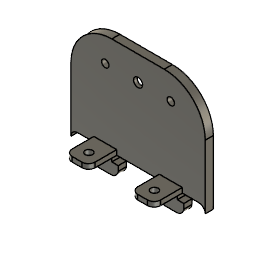
rodSupport (Autodesk Fusion 360 design; units mm, degrees)
part number: 2026-01-29-15-29-34-594
Autodesk Fusion 360 part; units mm, degrees
sketch "Sketch5" plane through (0, 0, 0) normal (0, 0, 1) x (1, 0, 0)
  line L0 (-41, -2.5) -> (41, -2.5)
  line L1 (41, -2.5) -> (41, 2.5)
  line L2 (41, 2.5) -> (-41, 2.5)
  line L3 (-41, 2.5) -> (-41, -2.5)
  line L4 (-41, -2.5) -> (41, 2.5) construction
  line L5 (41, -2.5) -> (-41, 2.5) construction
  line L6 (-37, 2.5) -> (-37, -2.5)
  line L7 (0, 2.5) -> (0, -2.5) construction
  line L8 (37, 2.5) -> (37, -2.5)
  line L9 (-10, -2.5) -> (10, -2.5) construction
  line L10 (23.95, -2.5) -> (16.05, -2.5)
  line L11 (16.05, -2.5) -> (16.05, 2.5)
  line L12 (16.05, 2.5) -> (23.95, 2.5)
  line L13 (23.95, 2.5) -> (23.95, -2.5)
  line L14 (-23.95, 2.5) -> (-23.95, -2.5)
  line L15 (-16.05, -2.5) -> (-16.05, 2.5)
  line L16 (-20, -2.5) -> (-20, 2.5) construction
  line L17 (20, -2.5) -> (20, 2.5) construction
  line L18 (-27, -2.5) -> (-13, -2.5)
  line L19 (-13, -2.5) -> (-13, -19.75)
  line L20 (-13, -19.75) -> (-27, -19.75)
  line L21 (-27, -19.75) -> (-27, -2.5)
  circle A0 centre (-20, -12.5) radius 2.25
  circle A1 centre (20, -12.5) radius 2.25
  line L22 (13, -19.75) -> (27, -19.75)
  line L23 (27, -19.75) -> (27, -2.5)
  line L24 (13, -2.5) -> (13, -19.75)
  dimension "d29" = 5
  dimension "d30" = 4
  dimension "d55" = 7.9
  dimension "d64" = 3.95
  dimension "d65" = 3.95
  dimension "d93" = 74
  dimension "d94" = 4
  dimension "d104" = 40
  dimension "d105" = 14
  dimension "d106" = 17.25
  dimension "d107" = 4.5
  dimension "d120" = 10
  constraint horizontal L0
  constraint perpendicular L0 L1
  constraint parallel L0 L2
  constraint parallel L1 L3
  constraint coincident L4 origin
  constraint coincident L5 origin
  constraint coincident L2 L6.start
  constraint coincident L0 L6.end
  constraint perpendicular L0 L6
  constraint midpoint L2 L7.start
  constraint midpoint L0 L7.end
  constraint symmetric L6.start L7 L8.start
  constraint symmetric L6.end L7 L8.end
  constraint horizontal L9
  constraint coincident L0 L9.start
  constraint horizontal L10
  constraint vertical L11
  constraint horizontal L12
  constraint vertical L13
  constraint coincident L0 L10.start
  constraint symmetric L7 L10.start L14.end
  constraint symmetric L7 L10.end L15.start
  constraint symmetric L7 L11.end L15.end
  constraint symmetric L7 L12.end L14.start
  constraint coincident L0 L16.start
  constraint coincident L2 L16.end
  constraint perpendicular L2 L16
  constraint symmetric L7 L16.start L17.start
  constraint symmetric L7 L16.end L17.end
  constraint coincident L2 L15.end
  constraint horizontal L18
  constraint vertical L19
  constraint horizontal L20
  constraint vertical L21
  constraint coincident L0 L18.start
  constraint midpoint L16.start L18
  constraint symmetric L7 L18.start L23.end
  constraint symmetric L7 L18.end L24.start
  constraint symmetric L7 L19.end L22.start
  constraint symmetric L7 L20.end L22.end
  constraint symmetric L7 A0 A1
  constraint vertical L16.start A0.centre
  measures "d29" distance of L0.end L1.end
  measures "d30" distance of L3 L6
  measures "d55" distance of L10.start L10.end
  measures "d64" distance of L14 L16
  measures "d65" distance of L15 L16
  measures "d93" distance of L6 L8
  measures "d94" distance of L1 L8
  measures "d104" distance of L16 L17
  measures "d105" distance of L18.start L18.end
  measures "d106" distance of L18.start L20.end
  measures "d107" diameter of A0
  measures "d120" distance of L18 A0.centre
sketch "Sketch6" plane through (0, 0, 0) normal (0, 1, 0) x (1, 0, 0)
  circle A0 centre (0, -45) radius 2.75
  line L0 (0, -56.6756) -> (0, 40) construction
  line L1 (-20, 40) -> (-20, 0) construction
  line L2 (20, 40) -> (20, 0) construction
  line L3 (20, 40) -> (20, 0) construction
  circle A1 centre (0, -45) radius 8.1
  line L4 (37.9681, -45) -> (-37.9681, -45) construction
  circle A2 centre (-20, -45) radius 2.25
  circle A3 centre (20, -45) radius 2.25
  point P0 (0, -45)
  point P1 (0, -60)
  point P2 (0, -56.6756)
  point P3 (0, 40)
  point P4 (-20, 16)
  point P5 (20, 16)
  point P6 (-20, 12)
  point P7 (-20, 5)
  point P8 (20, 16)
  point P9 (20, 5)
  point P10 (-20, 24)
  point P11 (20, 24)
  point P12 (-24.75, 0)
  point P13 (-37, 0)
  point P14 (20, 24)
  point P15 (20, 12)
  point P16 (37, 0)
  point P17 (20, 16)
  point P18 (24.75, 0)
  point P19 (20, 5)
  point P20 (0, -3)
  dimension "d35" = 5.5
  dimension "d36" = 40
  dimension "d45" = 20
  dimension "d46" = 20
  dimension "d48" = 40
  dimension "d49" = 12
  dimension "d50" = 5
  dimension "d51" = 16
  dimension "d52" = 8
  dimension "d53" = 16
  dimension "d54" = 12.25
  dimension "d77" = 15
  dimension "d99" = 16.2
  dimension "d103" = 45
  dimension "d108" = 3
  dimension "d115" = 4.5
  dimension "d116" = 20
  constraint vertical P1 L0.start
  constraint vertical P0 P1
  constraint coincident P0 A0.centre
  constraint coincident P2 L0.start
  constraint coincident P3 L0.end
  constraint vertical L0
  constraint horizontal P4 P17
  constraint horizontal P3 L1.start
  constraint vertical P4 L1.start
  constraint coincident L1 P6
  constraint coincident L1 P7
  constraint symmetric P4 L0 P17
  constraint symmetric L0 L1.start L2.start
  constraint symmetric L0 L1.end L2.end
  constraint symmetric L0 P7 P19
  constraint coincident L1 P10
  constraint symmetric L0 P10 P14
  constraint symmetric L0 P6 P15
  constraint symmetric L0 P12 P18
  constraint symmetric L0 P13 P16
  constraint concentric A0 A1
  constraint coincident L0 P20
  constraint horizontal L4
  constraint midpoint P0 L4
  constraint coincident L4 A2.centre
  constraint symmetric L0 A2 A3
  measures "d35" diameter of A0
  measures "d36" distance of P3 origin
  measures "d45" distance of P4 L0
  measures "d46" distance of P17 L0
  measures "d48" distance of L1.start L1.end
  measures "d49" distance of L1.end P6
  measures "d50" distance of L1.end P7
  measures "d51" distance of P4 L1.end
  measures "d52" distance of P4 P10
  measures "d53" distance of L1.start P10
  measures "d54" distance of P12 P13
  measures "d77" distance of P0 P1
  measures "d99" diameter of A1
  measures "d103" distance of P0 origin
  measures "d108" distance of origin P20
  measures "d115" diameter of A2
  measures "d116" distance of P0 A2.centre
extrude "Extrude10" add sketch "Sketch5" along normal up to surface (60 mm away) contours L0 L2 L3 L6 | L0 L2 L6 L14 L18 | L0 L2 L14 L15 L18 | L0 L2 L11 L15 L18 | L0 L2 L10 L11 L12 L13 | L0 L2 L8 L13 | L0 L1 L2 L8 makes body 1
extrude "Extrude14" add sketch "Sketch5" against normal up to surface (12 mm away) contours L0 L2 L14 L15 L18 bodies 1
sketch "Sketch8" plane through (-16.05, 0, 0) normal (1, 0, 0) x (0, 1, 0)
  line L0 (-2.5, -12) -> (2.5, -12)
  line L1 (2.5, -12) -> (2.5, 0)
  line L2 (2.5, 0) -> (-2.5, 0)
  line L3 (-2.5, 0) -> (-2.5, -12)
  line L4 (-2.5, -5) -> (2.5, -5)
  line L5 (2.5, -5) -> (-2.5, -5)
  point P0 (-2.5, 0)
  dimension "d59" = 5
  constraint coincident L3 L4.start
  constraint coincident L1 L4.end
  constraint perpendicular L1 L4
  measures "d59" distance of L4.start P0
extrude "Extrude15" add sketch "Sketch8" along normal blind 4 contours L0 L1 L3 L4 L5 bodies 1
fillet "Fillet1" radius 4 tangency weight 0.7 1 edges at (-12.05, 0, -12) on bodies 1
sketch "Sketch9" plane through (-23.95, 0, 0) normal (-1, 0, 0) x (0, -1, 0)
  line L0 (-2.5, -12) -> (2.5, -12)
  line L1 (2.5, -12) -> (2.5, 0)
  line L2 (2.5, 0) -> (-2.5, 0)
  line L3 (-2.5, 0) -> (-2.5, -12)
  line L4 (-2.5, -5) -> (2.5, -5)
  line L5 (-2.5, 0) -> (2.5, 0)
  dimension "d67" = 5
  constraint coincident L3 L4.start
  constraint coincident L1 L4.end
  constraint perpendicular L1 L4
  measures "d67" distance of L4 L5
extrude "Extrude16" add sketch "Sketch9" along normal blind 4 contours L0 L1 L3 L4 bodies 1
fillet "Fillet2" radius 4 tangency weight 0.7 1 edges at (-27.95, 0, -12) on bodies 1
split "Split1" by plane through (0, 0, 0) normal (0, 0, 1) bodies 1 makes body 2 at (-5.35, -2.5, 40)
mirror "Mirror1" about plane through (0, 0, 0) normal (1, 0, 0) of bodies 1 makes body 3
extrude "Extrude17" cut sketch "Sketch6" along normal up to surface (5 mm away) from surface at -2.5 contours A0 bodies 2
extrude "Extrude18" add sketch "Sketch5" against normal blind 4 contours L0 L2 L3 L6 bodies 2
pipe "Pipe1" cut diameter 8 along 1 edges at (-37, 0, -4) on bodies 2 bodies 2
extrude "Extrude19" add sketch "Sketch5" against normal blind 4 contours L0 L1 L2 L8 bodies 2
pipe "Pipe2" cut diameter 8 along 1 edges at (37, 0, -4) on bodies 2 bodies 2
extrude "Extrude20" cut sketch "Sketch6" against normal blind 2.8 from surface at 2.5 contours A1 bodies 2
extrude "Extrude21" add sketch "Sketch5" along normal up to surface (3 mm away) contours L0 L18 L19 L20 L21 | L0 L10 L22 L23 L24 bodies 1 2 3
fillet "Fillet3" radius 4 4 edges at (27, -19.75, 1.5) (13, -19.75, 1.5) (-13, -19.75, 1.5) (-27, -19.75, 1.5) on bodies 1
fillet "Fillet4" radius 25 2 edges at (41, 0, 60) (-41, 0, 60) on bodies 1
extrude "Extrude22" cut sketch "Sketch6" against normal up to surface (5 mm away) from surface at 2.5 contours A2 | A3 bodies 1
equation "d46 = d45"
equation "d47 = 8 mm"
equation "d51 = d48 / 2 - d47 / 2"
equation "d59 = d50"
equation "d67 = d50"
equation "d106 = d120 + d107 / 2 + 5 mm"
equation "d115 = d107"
